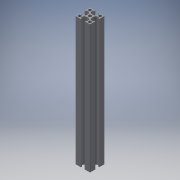
# Autodesk Inventor part: Profile
Saved by Autodesk Inventor 2016 (Build 200138000, 138)
## iProperties
Created: 2016-12-23
Part Number: Profile
Material: Generic
Document SubType Name: Modeling
Designer: inorn
Density: 1 g/cm^3
Appearance: Default
Author: inorn
Autodesk Inventor part; units mm, degrees
ref_plane "YZ Plane" through (0, 0, 0) normal (1, 0, 0) x (0, 1, 0)
ref_plane "XZ Plane" through (0, 0, 0) normal (0, 1, 0) x (-1, 0, 0)
ref_plane "XY Plane" through (0, 0, 0) normal (0, 0, 1) x (1, 0, 0)
sketch "Sketch1" plane through (0, 0, 0) normal (0, 0, 1) x (1, 0, 0)
  line L0 (-10, -10) -> (10, 10) construction
  line L1 (10, -10) -> (-10, 10) construction
  arc A0 (-10, -9.5) -> (-9.5, -10) centre (-9.5, -9.5) ccw
  arc A1 (-9.5, 10) -> (-10, 9.5) centre (-9.5, 9.5) ccw
  arc A2 (10, 9.5) -> (9.5, 10) centre (9.5, 9.5) ccw
  arc A3 (9.5, -10) -> (10, -9.5) centre (9.5, -9.5) ccw
  line L2 (7, -7) -> (-7, -7) construction
  line L3 (-7, -7) -> (-7, 7) construction
  line L4 (-7, 7) -> (7, 7) construction
  line L5 (7, 7) -> (7, -7) construction
  line L6 (7, -7) -> (-7, 7) construction
  line L7 (-7, -7) -> (7, 7) construction
  circle A4 centre (-7, -7) radius 2
  circle A5 centre (-7, 7) radius 2
  circle A6 centre (7, 7) radius 2
  circle A7 centre (7, -7) radius 2
  circle A8 centre (0, 0) radius 2.15
  line L8 (-8.5, 4.15) -> (-5.1906, 4.15)
  arc A9 (-5.1906, -4.15) -> (-5.1906, 4.15) centre (-8.8, 0) ccw
  line L9 (-5.1906, -4.15) -> (-8.5, -4.15)
  line L10 (-8.5, -4.15) -> (-8.5, -2.7559)
  line L11 (-8.5, 2.5441) -> (-8.5, 4.15)
  line L12 (-5.1906, -4.15) -> (-5.1906, 4.15) construction
  line L13 (-8.5, -2.7559) -> (-10, -2.7559)
  line L14 (-8.5, 2.5441) -> (-10, 2.5441)
  line L15 (-10, 9.5) -> (-10, 2.5441)
  line L16 (-10, -2.7559) -> (-10, -9.5)
  line L17 (4.15, -8.5) -> (2.7559, -8.5)
  line L18 (2.7559, -8.5) -> (2.7559, -10)
  line L19 (4.15, -5.1906) -> (-4.15, -5.1906) construction
  arc A10 (4.15, -5.1906) -> (-4.15, -5.1906) centre (0, -8.8) ccw
  line L20 (7, -7) -> (-7, 7) construction
  line L21 (10, -10) -> (-10, 10) construction
  line L22 (-4.15, -8.5) -> (-4.15, -5.1906)
  line L23 (4.15, -5.1906) -> (4.15, -8.5)
  line L24 (-2.5441, -8.5) -> (-2.5441, -10)
  line L25 (-2.5441, -8.5) -> (-4.15, -8.5)
  line L26 (8.5, 4.15) -> (8.5, 2.7559)
  line L27 (8.5, 2.7559) -> (10, 2.7559)
  line L28 (5.1906, 4.15) -> (5.1906, -4.15) construction
  arc A11 (5.1906, 4.15) -> (5.1906, -4.15) centre (8.8, 0) ccw
  line L29 (7, 7) -> (-7, -7) construction
  line L30 (10, 10) -> (-10, -10) construction
  line L31 (8.5, -4.15) -> (5.1906, -4.15)
  line L32 (5.1906, 4.15) -> (8.5, 4.15)
  line L33 (8.5, -2.5441) -> (10, -2.5441)
  line L34 (8.5, -2.5441) -> (8.5, -4.15)
  line L35 (-4.15, 8.5) -> (-2.7559, 8.5)
  line L36 (-2.7559, 8.5) -> (-2.7559, 10)
  line L37 (-4.15, 5.1906) -> (4.15, 5.1906) construction
  arc A12 (-4.15, 5.1906) -> (4.15, 5.1906) centre (0, 8.8) ccw
  line L38 (-7, 7) -> (7, -7) construction
  line L39 (-10, 10) -> (10, -10) construction
  line L40 (4.15, 8.5) -> (4.15, 5.1906)
  line L41 (-4.15, 5.1906) -> (-4.15, 8.5)
  line L42 (2.5441, 8.5) -> (2.5441, 10)
  line L43 (2.5441, 8.5) -> (4.15, 8.5)
  line L44 (-9.5, -10) -> (-2.5441, -10)
  line L45 (2.7559, -10) -> (9.5, -10)
  line L46 (9.5, 10) -> (2.5441, 10)
  line L47 (-2.7559, 10) -> (-9.5, 10)
  line L48 (10, -9.5) -> (10, -2.5441)
  line L49 (10, 2.7559) -> (10, 9.5)
  line L50 (2292.4151, 1187.1915) -> (2314.8128, 1187.1915)
  circle A13 centre (2303.6139, 1187.1915) radius 2.15
  line L51 (2307.7639, 1192.1343) -> (2307.7639, 1195.3915)
  arc A14 (2307.7639, 1195.3915) -> (2307.4639, 1195.6915) centre (2307.4639, 1195.3915) ccw
  line L52 (2307.4639, 1195.6915) -> (2306.5639, 1195.6915)
  arc A15 (2306.2639, 1195.9915) -> (2306.5639, 1195.6915) centre (2306.5639, 1195.9915) ccw
  line L53 (2306.2639, 1195.9915) -> (2306.2639, 1196.8915)
  arc A16 (2306.5639, 1197.1915) -> (2306.2639, 1196.8915) centre (2306.5639, 1196.8915) ccw
  line L54 (2306.5639, 1197.1915) -> (2313.3139, 1197.1915)
  arc A17 (2313.6139, 1196.8915) -> (2313.3139, 1197.1915) centre (2313.3139, 1196.8915) ccw
  line L55 (2313.6139, 1196.8915) -> (2313.6139, 1190.1415)
  arc A18 (2313.3139, 1189.8415) -> (2313.6139, 1190.1415) centre (2313.3139, 1190.1415) ccw
  line L56 (2313.3139, 1189.8415) -> (2312.4139, 1189.8415)
  arc A19 (2312.1139, 1190.1415) -> (2312.4139, 1189.8415) centre (2312.4139, 1190.1415) ccw
  line L57 (2312.1139, 1190.1415) -> (2312.1139, 1191.0415)
  arc A20 (2312.1139, 1191.0415) -> (2311.8139, 1191.3415) centre (2311.8139, 1191.0415) ccw
  line L58 (2311.8139, 1191.3415) -> (2308.5567, 1191.3415)
  arc A21 (2308.5567, 1191.3415) -> (2308.3217, 1191.2281) centre (2308.5567, 1191.0415) ccw
  arc A22 (2308.3217, 1191.2281) -> (2306.9212, 1187.4988) centre (2313.4048, 1187.1915) ccw
  line L59 (2306.9212, 1187.4988) -> (2306.6139, 1187.1915)
  line L60 (2306.6139, 1187.1915) -> (2306.9212, 1186.8843)
  arc A23 (2306.9212, 1186.8843) -> (2308.3217, 1183.155) centre (2313.4048, 1187.1915) ccw
  arc A24 (2308.3217, 1183.155) -> (2308.5567, 1183.0415) centre (2308.5567, 1183.3415) ccw
  line L61 (2308.5567, 1183.0415) -> (2311.8139, 1183.0415)
  arc A25 (2311.8139, 1183.0415) -> (2312.1139, 1183.3415) centre (2311.8139, 1183.3415) ccw
  line L62 (2312.1139, 1183.3415) -> (2312.1139, 1184.2415)
  arc A26 (2312.4139, 1184.5415) -> (2312.1139, 1184.2415) centre (2312.4139, 1184.2415) ccw
  line L63 (2312.4139, 1184.5415) -> (2313.3139, 1184.5415)
  arc A27 (2313.6139, 1184.2415) -> (2313.3139, 1184.5415) centre (2313.3139, 1184.2415) ccw
  line L64 (2313.6139, 1184.2415) -> (2313.6139, 1177.4915)
  arc A28 (2313.3139, 1177.1915) -> (2313.6139, 1177.4915) centre (2313.3139, 1177.4915) ccw
  line L65 (2313.3139, 1177.1915) -> (2306.5639, 1177.1915)
  arc A29 (2306.2639, 1177.4915) -> (2306.5639, 1177.1915) centre (2306.5639, 1177.4915) ccw
  line L66 (2306.2639, 1177.4915) -> (2306.2639, 1178.3915)
  arc A30 (2306.5639, 1178.6915) -> (2306.2639, 1178.3915) centre (2306.5639, 1178.3915) ccw
  line L67 (2306.5639, 1178.6915) -> (2307.4639, 1178.6915)
  arc A31 (2307.4639, 1178.6915) -> (2307.7639, 1178.9915) centre (2307.4639, 1178.9915) ccw
  line L68 (2307.7639, 1178.9915) -> (2307.7639, 1182.2488)
  arc A32 (2307.7639, 1182.2488) -> (2307.6505, 1182.4837) centre (2307.4639, 1182.2488) ccw
  arc A33 (2307.6505, 1182.4837) -> (2303.9212, 1183.8843) centre (2303.6139, 1177.4007) ccw
  line L69 (2303.9212, 1183.8843) -> (2303.6139, 1184.1915)
  line L70 (2303.6139, 1184.1915) -> (2303.3066, 1183.8843)
  arc A34 (2303.3066, 1183.8843) -> (2299.5774, 1182.4837) centre (2303.6139, 1177.4007) ccw
  arc A35 (2299.5774, 1182.4837) -> (2299.4639, 1182.2488) centre (2299.7639, 1182.2488) ccw
  line L71 (2299.4639, 1182.2488) -> (2299.4639, 1178.9915)
  arc A36 (2299.4639, 1178.9915) -> (2299.7639, 1178.6915) centre (2299.7639, 1178.9915) ccw
  line L72 (2299.7639, 1178.6915) -> (2300.6639, 1178.6915)
  arc A37 (2300.9639, 1178.3915) -> (2300.6639, 1178.6915) centre (2300.6639, 1178.3915) ccw
  line L73 (2300.9639, 1178.3915) -> (2300.9639, 1177.4915)
  arc A38 (2300.6639, 1177.1915) -> (2300.9639, 1177.4915) centre (2300.6639, 1177.4915) ccw
  line L74 (2300.6639, 1177.1915) -> (2293.9139, 1177.1915)
  arc A39 (2293.6139, 1177.4915) -> (2293.9139, 1177.1915) centre (2293.9139, 1177.4915) ccw
  line L75 (2293.6139, 1177.4915) -> (2293.6139, 1184.2415)
  arc A40 (2293.9139, 1184.5415) -> (2293.6139, 1184.2415) centre (2293.9139, 1184.2415) ccw
  line L76 (2293.9139, 1184.5415) -> (2294.8139, 1184.5415)
  arc A41 (2295.1139, 1184.2415) -> (2294.8139, 1184.5415) centre (2294.8139, 1184.2415) ccw
  line L77 (2295.1139, 1184.2415) -> (2295.1139, 1183.3415)
  arc A42 (2295.1139, 1183.3415) -> (2295.4139, 1183.0415) centre (2295.4139, 1183.3415) ccw
  line L78 (2295.4139, 1183.0415) -> (2298.6712, 1183.0415)
  arc A43 (2298.6712, 1183.0415) -> (2298.9061, 1183.155) centre (2298.6712, 1183.3415) ccw
  arc A44 (2298.9061, 1183.155) -> (2300.3066, 1186.8843) centre (2293.8231, 1187.1915) ccw
  line L79 (2300.3066, 1186.8843) -> (2300.6139, 1187.1915)
  line L80 (2300.6139, 1187.1915) -> (2300.3066, 1187.4988)
  arc A45 (2300.3066, 1187.4988) -> (2298.9061, 1191.2281) centre (2293.8231, 1187.1915) ccw
  arc A46 (2298.9061, 1191.2281) -> (2298.6712, 1191.3415) centre (2298.6712, 1191.0415) ccw
  line L81 (2298.6712, 1191.3415) -> (2295.4139, 1191.3415)
  arc A47 (2295.4139, 1191.3415) -> (2295.1139, 1191.0415) centre (2295.4139, 1191.0415) ccw
  line L82 (2295.1139, 1191.0415) -> (2295.1139, 1190.1415)
  arc A48 (2294.8139, 1189.8415) -> (2295.1139, 1190.1415) centre (2294.8139, 1190.1415) ccw
  line L83 (2294.8139, 1189.8415) -> (2293.9139, 1189.8415)
  arc A49 (2293.6139, 1190.1415) -> (2293.9139, 1189.8415) centre (2293.9139, 1190.1415) ccw
  line L84 (2293.6139, 1190.1415) -> (2293.6139, 1196.8915)
  arc A50 (2293.9139, 1197.1915) -> (2293.6139, 1196.8915) centre (2293.9139, 1196.8915) ccw
  line L85 (2293.9139, 1197.1915) -> (2300.6639, 1197.1915)
  arc A51 (2300.9639, 1196.8915) -> (2300.6639, 1197.1915) centre (2300.6639, 1196.8915) ccw
  line L86 (2300.9639, 1196.8915) -> (2300.9639, 1195.9915)
  arc A52 (2300.6639, 1195.6915) -> (2300.9639, 1195.9915) centre (2300.6639, 1195.9915) ccw
  line L87 (2300.6639, 1195.6915) -> (2299.7639, 1195.6915)
  arc A53 (2299.7639, 1195.6915) -> (2299.4639, 1195.3915) centre (2299.7639, 1195.3915) ccw
  line L88 (2299.4639, 1195.3915) -> (2299.4639, 1192.1343)
  arc A54 (2299.4639, 1192.1343) -> (2299.5774, 1191.8994) centre (2299.7639, 1192.1343) ccw
  arc A55 (2299.5774, 1191.8994) -> (2303.3066, 1190.4988) centre (2303.6139, 1196.9824) ccw
  line L89 (2303.3066, 1190.4988) -> (2303.6139, 1190.1915)
  line L90 (2303.6139, 1190.1915) -> (2303.9212, 1190.4988)
  arc A56 (2303.9212, 1190.4988) -> (2307.6505, 1191.8994) centre (2303.6139, 1196.9824) ccw
  arc A57 (2307.6505, 1191.8994) -> (2307.7639, 1192.1343) centre (2307.4639, 1192.1343) ccw
  line L91 (2294.1139, 1194.1915) -> (2299.1139, 1194.1915)
  line L92 (2296.6139, 1196.6915) -> (2296.6139, 1191.6915)
  circle A58 centre (2296.6139, 1194.1915) radius 2
  line L93 (2294.1139, 1180.1915) -> (2299.1139, 1180.1915)
  line L94 (2296.6139, 1177.6915) -> (2296.6139, 1182.6915)
  circle A59 centre (2296.6139, 1180.1915) radius 2
  line L95 (2303.6139, 1198.3904) -> (2303.6139, 1175.9927)
  line L96 (2313.1139, 1194.1915) -> (2308.1139, 1194.1915)
  line L97 (2310.6139, 1196.6915) -> (2310.6139, 1191.6915)
  circle A60 centre (2310.6139, 1194.1915) radius 2
  circle A61 centre (2310.6139, 1180.1915) radius 2
  line L98 (2310.6139, 1177.6915) -> (2310.6139, 1182.6915)
  line L99 (2313.1139, 1180.1915) -> (2308.1139, 1180.1915)
  point P0 (-10, 0)
  point P1 (-5.8595, 0)
  point P2 (-5.1906, 0)
  point P3 (-10, 0)
  point P4 (0, -5.8595)
  point P5 (0, -5.1906)
  point P6 (5.8595, 0)
  point P7 (5.1906, 0)
  point P8 (0, 5.8595)
  point P9 (0, 5.1906)
  dimension "d0" = 20
  dimension "d1" = 20
  dimension "d2" = 0.5
  dimension "d3" = 14
  dimension "d4" = 14
  dimension "d5" = 4
  dimension "d6" = 4.3
  dimension "d13" = 5.5
  dimension "d14" = 8.3
  dimension "d16" = 5.3
  dimension "d17" = 6.7
  dimension "d18" = 1.5
  dimension "d21" = 360
  constraints: 200 end point, 104 point on circle, 62 centre point, 16 tangent, 12 parallel, 10 perpendicular, 6 coincident, 6 equal radius, 5 midpoint, 4 horizontal, 1 collinear, 1 point on line, 1 vertical, 102 other
  measures "d0" distance of L1.end L0.end
  measures "d1" distance of L0.end L1.start
  measures "d2" radius of A0
  measures "d3" distance of L3.end L4.end
  measures "d4" distance of L2.end L3.end
  measures "d5" diameter of A4
  measures "d6" diameter of A8
  measures "d13" radius of A9
  measures "d14" distance between parallel lines of L8 L9
  measures "d16" distance between parallel lines of L14 L13
  measures "d18" distance of L11.start L14.end
extrude "Extrusion1" add sketch "Sketch1" along normal blind 176 contours L16 L13 L10 L9 A9 L8 L11 L14 L15 A1 L47 L36 L35 L41 A12 L40 L43 L42 L46 A2 L49 L27 L26 L32 A11 L31 L34 L33 L48 A3 L45 L18 L17 L23 A10 L22 L25 L24 L44 A0
body "Solid1"
